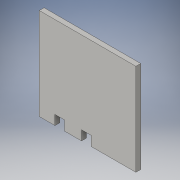
# Autodesk Inventor part: SideRWall
Saved by Autodesk Inventor 2016 (Build 200138000, 138)
## iProperties
Created: 2016-05-30
Part Number: SideRWall
Material: Generic
Document SubType Name: Modeling
Designer: cutrones
Density: 1 g/cm^3
Appearance: Default
Author: cutrones
Autodesk Inventor part; units mm, degrees
ref_plane "YZ Plane" through (0, 0, 0) normal (1, 0, 0) x (0, 1, 0)
ref_plane "XZ Plane" through (0, 0, 0) normal (0, 1, 0) x (-1, 0, 0)
ref_plane "XY Plane" through (0, 0, 0) normal (0, 0, 1) x (1, 0, 0)
sketch "Sketch1" plane through (0, 0, 0) normal (0, 0, 1) x (1, 0, 0)
  line L0 (0, 0) -> (254, 0)
  line L1 (254, 0) -> (254, 241.3)
  line L2 (254, 241.3) -> (0, 241.3)
  line L3 (0, 241.3) -> (0, 0)
  line L4 (88.9, 241.3) -> (88.9, 0)
  line L5 (41.275, 0) -> (66.675, 0)
  line L6 (66.675, 0) -> (66.675, 25.4)
  line L7 (66.675, 25.4) -> (41.275, 25.4)
  line L8 (41.275, 25.4) -> (41.275, 0)
  line L9 (111.125, 0) -> (136.525, 0)
  line L10 (136.525, 0) -> (136.525, 25.4)
  line L11 (136.525, 25.4) -> (111.125, 25.4)
  line L12 (111.125, 25.4) -> (111.125, 0)
  dimension "d0" = 254
  dimension "d1" = 241.3
  dimension "d2" = 88.9
  dimension "d3" = 25.4
  dimension "d4" = 25.4
  dimension "d5" = 25.4
  dimension "d6" = 22.225
  dimension "d7" = 22.225
  constraints: 26 end point, 6 parallel, 5 point on line, 4 perpendicular, 3 horizontal
  measures "d0" distance of L1.end L2.end
  measures "d1" distance of L0.end L1.end
  measures "d2" distance between parallel lines of L3 L4
  measures "d3" distance between parallel lines of L12 L10
  measures "d4" distance between parallel lines of L8 L6
  measures "d5" distance between parallel lines of L0 L7
  measures "d6" distance between parallel lines of L4 L6
  measures "d7" distance between parallel lines of L4 L12
extrude "Extrusion1" add sketch "Sketch1" along normal mid plane 12.7 contours L3 L2 L4 L0 L6 L7 L8 | L2 L1 L0 L10 L11 L12 L4
equation "\"d0\" = Width"
equation "\"d1\" = Height"
equation "\"d8\" = Thickness"
equation "\"Width\" = 254"
equation "\"Height\" = 241.3"
equation "\"Thickness\" = 12.7"
body "Solid1"
